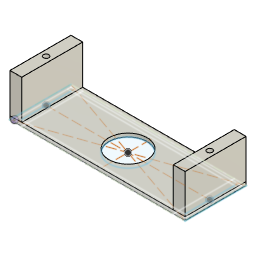
Cover (Autodesk Fusion 360 design; units mm, degrees)
Autodesk Fusion 360 part; units mm, degrees
sketch "Sketch1" plane through (0, 0, 0) normal (0, 0, 1) x (1, 0, 0)
  line L0 (0, 0) -> (100, 0)
  line L1 (100, 0) -> (100, 33)
  line L2 (100, 33) -> (0, 33)
  line L3 (0, 33) -> (0, 0)
  line L4 (0, 0) -> (2, 0) construction
  line L5 (2, 0) -> (2, 2) construction
  line L6 (2, 2) -> (0, 2) construction
  line L7 (0, 2) -> (0, 0) construction
  line L8 (0, 33) -> (2, 33) construction
  line L9 (2, 33) -> (2, 31) construction
  line L10 (2, 31) -> (0, 31) construction
  line L11 (0, 31) -> (0, 33) construction
  line L12 (100, 33) -> (98, 33) construction
  line L13 (98, 33) -> (98, 31) construction
  line L14 (98, 31) -> (100, 31) construction
  line L15 (100, 31) -> (100, 33) construction
  line L16 (100, 0) -> (98, 0) construction
  line L17 (98, 0) -> (98, 2) construction
  line L18 (98, 2) -> (100, 2) construction
  line L19 (100, 2) -> (100, 0) construction
  line L20 (98, 31) -> (98, 2)
  line L21 (98, 2) -> (2, 2)
  line L22 (2, 2) -> (2, 31)
  line L23 (98, 31) -> (2, 31)
  line L24 (2, 16.5) -> (98, 16.5) construction
  line L25 (50, 2) -> (50, 31) construction
  circle A0 centre (50, 16.5) radius 11.2
  line L26 (101.5, -1.5) -> (-1.5, -1.5) construction
  line L27 (-1.5, -1.5) -> (-1.5, 34.5) construction
  line L28 (-1.5, 34.5) -> (101.5, 34.5) construction
  line L29 (101.5, 34.5) -> (101.5, -1.5) construction
  line L30 (5.5, 33) -> (5.5, 0)
  line L31 (94.5, 33) -> (94.5, 0)
  circle A1 centre (2, 16.5) radius 1.6
  circle A2 centre (98, 16.5) radius 1.6
  line L32 (101.4, 34.4) -> (-1.4, 34.4)
  line L33 (-1.4, 34.4) -> (-1.4, -1.4)
  line L34 (-1.4, -1.4) -> (101.4, -1.4)
  line L35 (101.4, -1.4) -> (101.4, 34.4)
  line L36 (101.4, 34.4) -> (-1.4, -1.4) construction
  line L37 (-1.4, 34.4) -> (101.4, -1.4) construction
  line L38 (94.5, 33) -> (94.5, 34.4)
  line L39 (94.5, 0) -> (94.5, -1.4)
  line L40 (5.5, 0) -> (5.5, -1.4)
  line L41 (5.5, 33) -> (5.5, 34.4)
  point P0 (50, 16.5)
  point P1 (50, 16.5)
  dimension "d1" = 100
  dimension "d2" = 33
  dimension "d17" = 96
  dimension "d22" = 29
  dimension "d23" = 22.4
  dimension "d24" = 103
  dimension "d25" = 36
  dimension "d26" = 7
  dimension "d27" = 7
  dimension "d31" = 3.2
  dimension "d32" = 3.2
  dimension "d40" = 102.8
  dimension "d41" = 35.8
  constraint horizontal L0
  constraint vertical L1
  constraint horizontal L2
  constraint vertical L3
  constraint coincident L0.start L3.end
  constraint horizontal L4
  constraint vertical L5
  constraint horizontal L6
  constraint vertical L7
  constraint horizontal L8
  constraint vertical L9
  constraint horizontal L10
  constraint vertical L11
  constraint horizontal L12
  constraint vertical L13
  constraint horizontal L14
  constraint vertical L15
  constraint horizontal L16
  constraint vertical L17
  constraint horizontal L18
  constraint vertical L19
  constraint perpendicular L18 L20
  constraint perpendicular L5 L21
  constraint perpendicular L10 L22
  constraint perpendicular L22 L23
  constraint equal L13 L17
  constraint midpoint L22 L24.start
  constraint midpoint L20 L24.end
  constraint midpoint L21 L25.start
  constraint midpoint L23 L25.end
  constraint midpoint L25 P1
  constraint horizontal L26
  constraint perpendicular L26 L27
  constraint parallel L26 L28
  constraint parallel L27 L29
  constraint coincident P1 P0
  constraint coincident L2 L30.start
  constraint coincident L0 L30.end
  constraint perpendicular L0 L30
  constraint coincident L2 L31.start
  constraint coincident L0 L31.end
  constraint perpendicular L0 L31
  constraint coincident L24.start A1.centre
  constraint coincident L24.end A2.centre
  constraint horizontal L32
  constraint perpendicular L32 L33
  constraint parallel L32 L34
  constraint parallel L33 L35
  constraint coincident L36 P1
  constraint coincident L37 P1
  constraint coincident L32 L38.end
  constraint perpendicular L32 L38
  constraint coincident L34 L39.end
  constraint perpendicular L34 L39
  constraint coincident L34 L40.end
  constraint perpendicular L34 L40
  constraint coincident L32 L41.end
  constraint perpendicular L32 L41
  measures "d1" distance of L0.start L0.end
  measures "d2" distance of L0.start L2.end
  measures "d17" distance of L9.end L13.end
  measures "d22" distance of L13.end L17.end
  measures "d23" diameter of A0
  measures "d24" distance of L27.end L28.end
  measures "d25" distance of L26.end L27.end
  measures "d26" distance of L27 L30
  measures "d27" distance of L29 L31
  measures "d31" diameter of A1
  measures "d32" diameter of A2
  measures "d40" distance of L33.end L34.end
  measures "d41" distance of L32.end L33.end
extrude "Extrude5" add sketch "Sketch1" along normal blind 2 contours L0 L2 L3 L21 L22 L23 L30 A1 | L0 L2 L3 L32 L33 L34 L40 L41 | L0 L21 L30 L31 | L0 L34 L39 L40 | L0 L1 L2 L20 L21 L23 L31 A2 | L0 L1 L2 L32 L34 L35 L38 L39 | L21 L23 L30 L31 | L21 L22 L23 L30 A1 | L2 L32 L38 L41 | L2 L23 L30 L31 | L20 L21 L23 L31 A2 makes body 1
extrude "Extrude6" add sketch "Sketch1" along normal blind 23 from surface at 2 separate body contours L0 L2 L3 L21 L22 L23 L30 A1 | L0 L2 L3 L32 L33 L34 L40 L41 | L0 L1 L2 L20 L21 L23 L31 A2 | L0 L1 L2 L32 L34 L35 L38 L39 | L21 L22 L23 L30 A1 | L20 L21 L23 L31 A2 makes body 2 at (-1.4, 22.4667, 9.6667) makes body 3 at (101.4, 10.5333, 9.6667)
